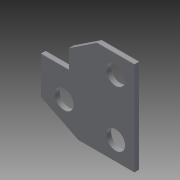
# Autodesk Inventor part: P1-7
Saved by Autodesk Inventor 2014 (Build 180170000, 170)
## iProperties
Created: 2017-02-06
Part Number: P1-7
Material: Generic
Document SubType Name: Modeling
Designer: mschaffel
Density: 1 g/cm^3
Appearance: Default
Author: mschaffel
Autodesk Inventor part; units mm, degrees
ref_plane "YZ Plane" through (0, 0, 0) normal (1, 0, 0) x (0, 1, 0)
ref_plane "XZ Plane" through (0, 0, 0) normal (0, 1, 0) x (-1, 0, 0)
ref_plane "XY Plane" through (0, 0, 0) normal (0, 0, 1) x (1, 0, 0)
sketch "Sketch1" plane through (0, 0, 0) normal (0, 1, 0) x (-1, 0, 0)
  line L0 (0, 0) -> (0, 100)
  line L1 (0, 100) -> (40, 100)
  line L2 (0, 0) -> (60, 0)
  line L3 (100, 20) -> (60, 0)
  line L4 (100, 20) -> (100, 60)
  circle A0 centre (20, 20) radius 10
  line L5 (100, 60) -> (70, 60)
  line L6 (70, 60) -> (70, 80)
  line L7 (70, 80) -> (40, 100)
  circle A1 centre (75, 30) radius 10
  circle A2 centre (20, 80) radius 10
  dimension "d0" = 100
  dimension "d1" = 40
  constraints: 16 end point, 3 centre point, 1 parallel, 1 perpendicular, 1 vertical
  measures "d0" distance of L0.start L0.end
  measures "d1" distance of L0.end L1.end
extrude "Extrusion1" add sketch "Sketch1" along normal blind 5
body "Solid1"
